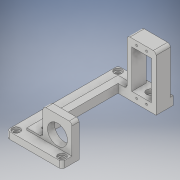
# Autodesk Inventor part: Cuerpo - Acople Hombro
Saved by Autodesk Inventor 2019 (Build 230136000, 136)
## iProperties
Created: 2020-03-08
Part Number: Cuerpo - Acople Hombro
Material: Genérico
Document SubType Name: Modeling
Designer: eddysanoli
Density: 1 g/cm^3
Appearance: Valor por defecto
Author: eddysanoli
Autodesk Inventor part; units mm, degrees
ref_plane "YZ Plane" through (0, 0, 0) normal (1, 0, 0) x (0, 1, 0)
ref_plane "XZ Plane" through (0, 0, 0) normal (0, 1, 0) x (-1, 0, 0)
ref_plane "XY Plane" through (0, 0, 0) normal (0, 0, 1) x (1, 0, 0)
sketch "Boceto1" plane through (0, 0, 0) normal (0, 1, 0) x (-1, 0, 0)
  line L0 (0, 0) -> (0, 18)
  line L1 (0, 18) -> (58.0941, 18)
  line L2 (58.0941, 18) -> (58.0941, -99.05)
  line L3 (58.0941, -99.05) -> (0, -99.05)
  line L4 (0, -99.05) -> (0, -81.05)
  line L5 (0, -81.05) -> (40.0941, -81.05)
  line L6 (40.0941, -81.05) -> (40.0941, 0)
  line L7 (40.0941, 0) -> (0, 0)
  dimension "d0" = 81.05
  dimension "d1" = 18
  dimension "d2" = 18
  dimension "d3" = 40.0941
  constraints: 16 end point, 6 perpendicular, 2 point on line, 1 collinear, 1 vertical
  measures "d0" distance of L5.end L6.end
  measures "d1" distance between parallel lines of L2 L6
  measures "d2" distance of L0.start L0.end
  measures "d3" distance of L6.end L0.start
extrude "Extrusión1" add sketch "Boceto1" along normal blind 4
sketch "Boceto2" plane through (0, 4, 0) normal (0, 1, 0) x (1, 0, 0)
  line L0 (0, -18) -> (0, 0) projected
  line L1 (0, 0) -> (-30.5, 0)
  line L2 (-30.5, 0) -> (-30.5, -7.5)
  line L3 (-30.5, -7.5) -> (0, -7.5)
  line L4 (0, -7.5) -> (0, 0)
  point P0 (0, 81.05)
  dimension "d6" = 30.5
  dimension "d7" = 7.5
  constraints: 8 end point, 2 parallel, 1 horizontal, 1 perpendicular
  measures "d6" distance between parallel lines of L0 L2
  measures "d7" distance between parallel lines of L1 L3
sketch "Boceto3" plane through (0, 4, 0) normal (0, 1, 0) x (1, 0, 0)
  line L0 (0, 81.05) -> (-30.5, 81.05)
  line L1 (-30.5, 81.05) -> (-30.5, 96.05)
  line L2 (-30.5, 96.05) -> (0, 96.05)
  line L3 (0, 96.05) -> (0, 81.05)
  line L4 (-30.5, 0) -> (-30.5, -7.5) projected
  point P0 (0, 0)
  dimension "d9" = 15
  dimension "d21" = 30.5
  constraints: 8 end point, 2 parallel, 1 horizontal, 1 perpendicular
  measures "d9" distance between parallel lines of L2 L0
  measures "d21" distance of L0.start L0.end
extrude "Extrusión2" add sketch "Boceto3" along normal blind 50.5
sketch "Boceto4" plane through (-40.0941, 0, -81.05) normal (0, 0, 1) x (1, 0, 0)
  line L0 (14.5941, 46.5) -> (35.0941, 46.5)
  line L1 (35.0941, 46.5) -> (35.0941, 6)
  line L2 (35.0941, 6) -> (14.5941, 6)
  line L3 (14.5941, 6) -> (14.5941, 46.5)
  line L4 (40.0941, 0) -> (0, 0) projected
  line L5 (40.0941, 0) -> (40.0941, 54.5) projected
  line L6 (9.5941, 54.5) -> (40.0941, 54.5) projected
  line L7 (9.5941, 4) -> (9.5941, 54.5) projected
  line L8 (0, 4) -> (9.5941, 4) projected
  line L9 (0, 0) -> (0, 4) projected
  circle A0 centre (19.5941, 2.05) radius 1
  circle A1 centre (30.0941, 2.05) radius 1
  circle A2 centre (19.5941, 50.45) radius 1
  circle A3 centre (30.0941, 50.45) radius 1
  dimension "d12" = 40.5
  dimension "d13" = 20.5
  dimension "d14" = 2
  dimension "d15" = 3.95
  dimension "d16" = 3.95
  dimension "d17" = 5
  dimension "d18" = 5
  dimension "d19" = 2.05
  dimension "d20" = 5
  dimension "d22" = 30.5
  dimension "d23" = 54.5
  dimension "d24" = 48.4
  constraints: 8 end point, 4 centre point, 3 equal radius, 2 horizontal alignment, 2 parallel, 2 vertical alignment, 1 horizontal, 1 perpendicular
  measures "d12" distance of L0.end L1.end
  measures "d13" distance of L1.end L2.end
  measures "d14" diameter of A2
  measures "d15" distance from line of L0 A3.centre
  measures "d16" distance from line of L2 A0.centre
  measures "d17" distance from line of L3 A2.centre
  measures "d18" distance from line of L1 A3.centre
  measures "d19" distance from line of L4 A1.centre
  measures "d20" distance between parallel lines of L5 L1
  measures "d22" distance of L6.start L5.end
  measures "d23" distance between parallel lines of L4 L6
  measures "d24" distance of A0.centre A2.centre
sketch "Boceto5" plane through (-40.0941, 0, -81.05) normal (0, 0, 1) x (1, 0, 0)
  circle A0 centre (19.5941, 50.45) radius 1 projected
  circle A1 centre (30.0941, 50.45) radius 1 projected
  circle A2 centre (19.5941, 2.05) radius 1 projected
  circle A3 centre (30.0941, 2.05) radius 1 projected
  point P0 (40.0941, 0)
extrude "Extrusión3" cut sketch "Boceto4" against normal up to surface (15 mm away) contours L0 L1 L2 L3
extrude "Extrusión4" cut sketch "Boceto5" against normal up to surface (15 mm away)
extrude "Extrusión5" add sketch "Boceto2" along normal blind 30.5
ref_plane "Plano de trabajo2" through (-25.5, 6, -88.55) normal (0, 1, 0) x (1, 0, 0)
sketch "Boceto6" plane through (0, 0, 0) normal (0, 0, -1) x (-1, 0, 0)
  circle A0 centre (15.25, 16.1) radius 10.5
  line L0 (0, 34.5) -> (30.5, 34.5) projected
  point P0 (0, 0)
  point P1 (0, 6)
  point P2 (15.25, 34.5)
  dimension "d31" = 10.1
  dimension "d32" = 21
  constraints: 1 centre point, 1 midpoint, 1 vertical alignment
  measures "d31" vertical distance of point (0, 6) A0.centre
  measures "d32" diameter of A0
extrude "Extrusión6" cut sketch "Boceto6" against normal up to surface (7.5 mm away)
sketch "Boceto7" plane through (0, 4, -96.05) normal (0, 0, -1) x (-1, 0, 0)
  line L0 (0, 0) -> (58.0941, 0) projected
  line L1 (30.5, 0) -> (30.5, 50.5) projected
  line L2 (0, 0) -> (30.5, 0)
  line L3 (30.5, 0) -> (30.5, 2)
  line L4 (30.5, 2) -> (0, 2)
  line L5 (0, 2) -> (0, 0)
  line L6 (25.5, 2) -> (5, 2) projected
  point P0 (0, -4)
  constraints: 8 end point, 2 parallel, 2 point on line, 1 horizontal, 1 perpendicular
extrude "Extrusión7" add sketch "Boceto7" along normal up to surface (3 mm away)
sketch "Boceto8" plane through (0, 4, 0) normal (0, 1, 0) x (1, 0, 0)
  line L0 (-30.5, -7.5) -> (-30.5, 0) projected
  line L1 (-30.5, 0) -> (-30.5, -7.5)
  line L2 (-30.5, -7.5) -> (-47.5941, -7.5)
  line L3 (-47.5941, -7.5) -> (-47.5941, 88.55)
  line L4 (-47.5941, 88.55) -> (-30.5, 88.55)
  line L5 (-30.5, 81.05) -> (-30.5, 99.05) projected
  line L6 (-30.5, 88.55) -> (-30.5, 81.05)
  line L7 (-40.0941, 81.05) -> (-30.5, 81.05) projected
  line L8 (-30.5, 81.05) -> (-40.0941, 81.05)
  line L9 (-40.0941, 0) -> (-40.0941, 81.05) projected
  line L10 (-40.0941, 81.05) -> (-40.0941, 0)
  line L11 (-40.0941, 0) -> (-30.5, 0)
  line L12 (-40.0941, 0) -> (0, 0) projected
  dimension "d38" = 7.5
  dimension "d39" = 7.5
  dimension "d40" = 7.5
  constraints: 16 end point, 5 collinear, 3 perpendicular, 1 point on line
  measures "d38" distance of L0.start L0.end
  measures "d39" distance between parallel lines of L7 L4
  measures "d40" distance between parallel lines of L3 L9
extrude "Extrusión8" add sketch "Boceto8" along normal up to surface (2 mm away)
fillet "Empalme2" radius 3 10 edges at (-30.5, 54.5, -88.55) (0, 54.5, -88.55) (-30.5, 6, 3.75) (-30.5, 6, -84.8) (-30.5, 4, -93.8) (-30.5, 34.5, 3.75) (0, 34.5, 3.75) (0, 2, 18) (-58.0941, 2, -99.05) (-58.0941, 2, 18)
sketch "Boceto9" plane through (0, 4, 0) normal (0, 1, 0) x (1, 0, 0)
  circle A0 centre (-5, -13) radius 2.35
  circle A1 centre (-53.0941, -13) radius 2.35
  circle A2 centre (-53.0941, 94.05) radius 2.35
  arc A3 (-58.0941, -15) -> (-55.0941, -18) centre (-55.0941, -15) ccw projected
  arc A4 (-55.0941, 99.05) -> (-58.0941, 96.05) centre (-55.0941, 96.05) ccw projected
  line L0 (-58.0941, 96.05) -> (-58.0941, -15) projected
  line L1 (-33.5, 99.05) -> (-55.0941, 99.05) projected
  line L2 (-55.0941, -18) -> (-3, -18) projected
  line L3 (0, -15) -> (0, -7.5) projected
  circle A5 centre (-15.25, 90.05) radius 2.35
  line L4 (-5, 81.05) -> (-25.5, 81.05) projected
  line L5 (0, 99.05) -> (0, 81.05) projected
  point P0 (0, 0)
  point P1 (-15.25, 81.05)
  point P2 (0, 90.05)
  dimension "d48" = 5
  dimension "d49" = 5
  dimension "d50" = 4.7
  dimension "d51" = 5
  dimension "d52" = 5
  constraints: 4 centre point, 3 equal radius, 2 horizontal alignment, 2 midpoint, 2 vertical alignment
  measures "d48" distance from line of L0 A2.centre
  measures "d49" distance from line of L1 A2.centre
  measures "d50" diameter of A2
  measures "d51" distance from line of L2 A0.centre
  measures "d52" distance from line of L3 A0.centre
extrude "Extrusion10" cut sketch "Boceto9" along normal mid plane 10
sketch "Sketch10" plane through (0, 4, 0) normal (0, 1, 0) x (1, 0, 0)
  circle A0 centre (-5, -13) radius 2.35 projected
  circle A1 centre (-5, -13) radius 4.05
  circle A2 centre (-53.0941, -13) radius 2.35 projected
  circle A3 centre (-53.0941, -13) radius 4.05
  circle A4 centre (-53.0941, 94.05) radius 2.35 projected
  circle A5 centre (-53.0941, 94.05) radius 4.05
  circle A6 centre (-15.25, 90.05) radius 2.35 projected
  circle A7 centre (-15.25, 90.05) radius 4.3063
  point P0 (0, 0)
  dimension "d55" = 8.1
  constraints: 4 centre point, 4 coincident, 2 equal radius
  measures "d55" diameter of A1
extrude "Extrusion11" cut sketch "Sketch10" against normal blind 2 contours A1 | A3 | A5
sketch "Sketch11" plane through (-25.5, 6, -81.05) normal (0, 1, 0) x (1, 0, 0)
  circle A0 centre (10.25, 9) radius 2.35 projected
  circle A1 centre (10.25, 9) radius 4.05
  circle A2 centre (-27.5941, 13) radius 4.05 projected
  point P0 (25.5, -81.05)
  constraints: 1 centre point, 1 coincident, 1 equal radius
extrude "Extrusion12" cut sketch "Sketch11" against normal blind 4.5 contours A1
sketch "Sketch12" plane through (0, 0, 0) normal (0, -1, 0) x (1, 0, 0)
  circle A0 centre (-53.0941, -94.05) radius 2.35 projected
  circle A1 centre (-5, 13) radius 2.35 projected
  circle A2 centre (-53.0941, 13) radius 2.35 projected
  circle A3 centre (-15.25, -90.05) radius 2.35 projected
  arc A4 (-55.0941, 18) -> (-58.0941, 15) centre (-55.0941, 15) ccw projected
  line L0 (-58.0941, 15) -> (-58.0941, -96.05) projected
  arc A5 (-58.0941, -96.05) -> (-55.0941, -99.05) centre (-55.0941, -96.05) ccw projected
  line L1 (-55.0941, -99.05) -> (0, -99.05) projected
  line L2 (0, -99.05) -> (0, -81.05) projected
  line L3 (0, -81.05) -> (-40.0941, -81.05) projected
  line L4 (-40.0941, -81.05) -> (-40.0941, 0) projected
  line L5 (-40.0941, 0) -> (0, 0) projected
  line L6 (0, 0) -> (0, 15) projected
  arc A6 (0, 15) -> (-3, 18) centre (-3, 15) ccw projected
  line L7 (-3, 18) -> (-55.0941, 18) projected
extrude "Extrusion13" add sketch "Sketch12" along normal blind 3
equation "\"d1\" = d2"
equation "\"d6\" = d21"
equation "\"d9\" = 2 * d7"
equation "\"d12\" = largo_servo"
equation "\"d13\" = ancho_servo"
equation "\"d16\" = d15"
equation "\"d18\" = d17"
equation "\"d19\" = -0.5 * d24 - 0.5 * d14 + 0.5 * d23"
equation "\"d20\" = -0.5 * ancho_servo + 0.5 * d22"
equation "\"d29\" = d6"
equation "\"d33\" = d6"
equation "\"d35\" = d6"
equation "\"d39\" = d38"
equation "\"d40\" = d39"
equation "\"d41\" = d6"
equation "\"d51\" = d49"
equation "\"d52\" = d48"
equation "\"largo_servo\" = 40.5"
equation "\"ancho_servo\" = 20.5"
